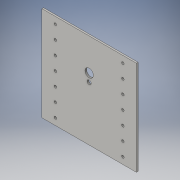
# Autodesk Inventor part: ClawPlate
Saved by Autodesk Inventor 2016 (Build 200138000, 138)
## iProperties
Created: 2016-01-25
Part Number: ClawPlate
Material: Generic
Document SubType Name: Modeling
Designer: Mentor1102
Density: 1 g/cm^3
Appearance: Default
Author: Mentor1102
Autodesk Inventor part; units mm, degrees
ref_plane "YZ Plane" through (0, 0, 0) normal (1, 0, 0) x (0, 1, 0)
ref_plane "XZ Plane" through (0, 0, 0) normal (0, 1, 0) x (-1, 0, 0)
ref_plane "XY Plane" through (0, 0, 0) normal (0, 0, 1) x (1, 0, 0)
sketch "Sketch1" plane through (0, 0, 0) normal (0, 0, 1) x (1, 0, 0)
  line L0 (0, 0) -> (177.8, 0)
  line L1 (177.8, 0) -> (177.8, 177.8)
  line L2 (177.8, 177.8) -> (0, 177.8)
  line L3 (0, 177.8) -> (0, 0)
  dimension "d0" = 177.8
  dimension "d1" = 177.8
  constraints: 8 end point, 2 parallel, 1 horizontal, 1 perpendicular
  measures "d0" distance of L2.end L1.end
  measures "d1" distance of L1.end L0.end
extrude "Extrusion1" add sketch "Sketch1" along normal blind 3.175
sketch "Sketch2" plane through (0, 0, 3.175) normal (0, 0, 1) x (1, 0, 0)
  line L0 (0, 0) -> (177.8, 0) projected
  line L1 (177.8, 0) -> (177.8, 177.8) projected
  line L2 (177.8, 177.8) -> (0, 177.8) construction
  line L3 (0, 177.8) -> (0, 0) projected
  line L4 (177.8, 177.8) -> (0, 177.8) construction
  line L5 (88.9, 177.8) -> (76.2, 177.8) construction
  line L6 (88.9, 177.8) -> (101.6, 177.8) construction
  line L7 (76.2, 177.8) -> (76.2, 127) construction
  line L8 (76.2, 127) -> (101.6, 127) construction
  line L9 (101.6, 177.8) -> (101.6, 127) construction
  line L10 (88.9, 127) -> (88.9, 107.95) construction
  circle A0 centre (88.9, 117.475) radius 9.525 construction
  circle A1 centre (88.9, 117.475) radius 7.874
  dimension "d4" = 12.7
  dimension "d5" = 12.7
  dimension "d6" = 50.8
  dimension "d7" = 19.05
  dimension "d8" = 15.748
  constraints: 12 end point, 3 midpoint, 3 vertical, 2 point on line, 1 centre point, 1 coincident, 1 perpendicular, 1 vertical alignment, 2 other
  measures "d4" distance of L5.start L5.end
  measures "d5" distance of L5.start L6.end
  measures "d6" distance of L5.end L7.end
  measures "d7" distance of L10.start L10.end
  measures "d8" diameter of A1
extrude "Extrusion2" cut sketch "Sketch2" against normal through all
sketch "Sketch3" plane through (0, 0, 3.175) normal (0, 0, 1) x (1, 0, 0)
  circle A0 centre (88.9, 117.475) radius 7.874 projected
  line L0 (0, 0) -> (177.8, 0) projected
  line L1 (177.8, 0) -> (177.8, 177.8) projected
  line L2 (177.8, 177.8) -> (0, 177.8) projected
  line L3 (0, 177.8) -> (0, 0) projected
  circle A1 centre (88.9, 117.475) radius 10.16 construction
  line L4 (88.9, 117.475) -> (88.9, 107.315) construction
  line L5 (88.9, 107.315) -> (88.9, 102.235) construction
  circle A2 centre (88.9, 102.235) radius 3.9116
  dimension "d11" = 20.32
  dimension "d12" = 5.08
  dimension "d13" = 7.8232
  constraints: 4 end point, 2 coincident, 2 vertical, 1 centre point, 1 vertical alignment, 2 other
  measures "d12" distance of L4.end L5.end
  measures "d13" diameter of A2
extrude "Extrusion3" cut sketch "Sketch3" against normal through all contours A2
sketch "Sketch4" plane through (0, 0, 3.175) normal (0, 0, 1) x (1, 0, 0)
  circle A0 centre (88.9, 102.235) radius 3.9116 projected
  circle A1 centre (88.9, 117.475) radius 7.874 projected
  line L0 (0, 0) -> (177.8, 0) projected
  line L1 (177.8, 0) -> (177.8, 177.8) projected
  line L2 (177.8, 177.8) -> (0, 177.8) construction
  line L3 (0, 177.8) -> (0, 0) projected
  line L4 (0, 177.8) -> (25.4, 177.8) construction
  line L5 (177.8, 177.8) -> (0, 177.8) construction
  line L6 (177.8, 177.8) -> (152.4, 177.8) construction
  line L7 (25.4, 177.8) -> (25.4, 152.4) construction
  line L8 (152.4, 177.8) -> (152.4, 152.4) construction
  circle A2 centre (25.4, 152.4) radius 2.3812
  circle A3 centre (152.4, 152.4) radius 2.3813
  line L9 (0, 165.1) -> (25.4, 165.1) construction
  line L10 (177.8, 165.1) -> (152.4, 165.1) construction
  line L11 (25.4, 165.1) -> (25.4, 139.7) construction
  line L12 (152.4, 165.1) -> (152.4, 139.7) construction
  circle A4 centre (25.4, 139.7) radius 2.3812
  line L13 (0, 152.4) -> (25.4, 152.4) construction
  line L14 (177.8, 152.4) -> (152.4, 152.4) construction
  line L15 (25.4, 152.4) -> (25.4, 127) construction
  line L16 (152.4, 152.4) -> (152.4, 127) construction
  circle A5 centre (25.4, 127) radius 2.3812
  line L17 (0, 139.7) -> (25.4, 139.7) construction
  line L18 (177.8, 139.7) -> (152.4, 139.7) construction
  line L19 (25.4, 139.7) -> (25.4, 114.3) construction
  line L20 (152.4, 139.7) -> (152.4, 114.3) construction
  circle A6 centre (25.4, 114.3) radius 2.3812
  line L21 (0, 127) -> (25.4, 127) construction
  line L22 (177.8, 127) -> (152.4, 127) construction
  line L23 (25.4, 127) -> (25.4, 101.6) construction
  line L24 (152.4, 127) -> (152.4, 101.6) construction
  circle A7 centre (25.4, 101.6) radius 2.3812
  line L25 (0, 114.3) -> (25.4, 114.3) construction
  line L26 (177.8, 114.3) -> (152.4, 114.3) construction
  line L27 (25.4, 114.3) -> (25.4, 88.9) construction
  line L28 (152.4, 114.3) -> (152.4, 88.9) construction
  circle A8 centre (25.4, 88.9) radius 2.3812
  line L29 (0, 101.6) -> (25.4, 101.6) construction
  line L30 (177.8, 101.6) -> (152.4, 101.6) construction
  line L31 (25.4, 101.6) -> (25.4, 76.2) construction
  line L32 (152.4, 101.6) -> (152.4, 76.2) construction
  circle A9 centre (25.4, 76.2) radius 2.3812
  line L33 (0, 88.9) -> (25.4, 88.9) construction
  line L34 (177.8, 88.9) -> (152.4, 88.9) construction
  line L35 (25.4, 88.9) -> (25.4, 63.5) construction
  line L36 (152.4, 88.9) -> (152.4, 63.5) construction
  circle A10 centre (25.4, 63.5) radius 2.3812
  line L37 (0, 76.2) -> (25.4, 76.2) construction
  line L38 (177.8, 76.2) -> (152.4, 76.2) construction
  line L39 (25.4, 76.2) -> (25.4, 50.8) construction
  line L40 (152.4, 76.2) -> (152.4, 50.8) construction
  circle A11 centre (25.4, 50.8) radius 2.3812
  line L41 (0, 63.5) -> (25.4, 63.5) construction
  line L42 (177.8, 63.5) -> (152.4, 63.5) construction
  line L43 (25.4, 63.5) -> (25.4, 38.1) construction
  line L44 (152.4, 63.5) -> (152.4, 38.1) construction
  circle A12 centre (25.4, 38.1) radius 2.3812
  line L45 (0, 50.8) -> (25.4, 50.8) construction
  line L46 (177.8, 50.8) -> (152.4, 50.8) construction
  line L47 (25.4, 50.8) -> (25.4, 25.4) construction
  line L48 (152.4, 50.8) -> (152.4, 25.4) construction
  circle A13 centre (25.4, 25.4) radius 2.3812
  line L49 (0, 38.1) -> (25.4, 38.1) construction
  line L50 (177.8, 38.1) -> (152.4, 38.1) construction
  line L51 (25.4, 38.1) -> (25.4, 12.7) construction
  line L52 (152.4, 38.1) -> (152.4, 12.7) construction
  circle A14 centre (25.4, 12.7) radius 2.3812
  circle A15 centre (152.4, 139.7) radius 2.3813
  circle A16 centre (152.4, 127) radius 2.3813
  circle A17 centre (152.4, 114.3) radius 2.3813
  circle A18 centre (152.4, 101.6) radius 2.3813
  circle A19 centre (152.4, 88.9) radius 2.3813
  circle A20 centre (152.4, 76.2) radius 2.3813
  circle A21 centre (152.4, 63.5) radius 2.3813
  circle A22 centre (152.4, 50.8) radius 2.3813
  circle A23 centre (152.4, 38.1) radius 2.3813
  circle A24 centre (152.4, 25.4) radius 2.3813
  circle A25 centre (152.4, 12.7) radius 2.3813
  circle A26 centre (25.4, 165.1) radius 2.3813
  circle A27 centre (152.4, 165.1) radius 2.3812
  dimension "d16" = 25.4
  dimension "d17" = 25.4
  dimension "d18" = 25.4
  dimension "d19" = 25.4
  dimension "d20" = 4.7625
  dimension "d21" = 4.7625
  dimension "d24" = 12.7
  dimension "d31" = 12.7
  dimension "d47" = 4.7625
  dimension "d48" = 4.7625
  constraints: 96 end point, 26 centre point, 17 coincident, 4 vertical, 2 point on line, 154 other
  measures "d16" distance of L2.end L4.end
  measures "d17" distance of L1.end L6.end
  measures "d18" distance of L4.end L7.end
  measures "d19" distance of L6.end L8.end
  measures "d20" diameter of A2
  measures "d21" diameter of A3
  measures "d24" distance of L4.end L9.end
  measures "d31" distance of A3.centre A15.centre
  measures "d47" diameter of A26
  measures "d48" diameter of A27
sketch "Sketch5" plane through (0, 0, 3.175) normal (0, 0, 1) x (1, 0, 0)
  circle A0 centre (88.9, 102.235) radius 3.9116 construction
  circle A1 centre (88.9, 117.475) radius 7.874 construction
  line L0 (0, 0) -> (177.8, 0) construction
  line L1 (177.8, 0) -> (177.8, 177.8) construction
  line L2 (177.8, 177.8) -> (0, 177.8) construction
  line L3 (0, 177.8) -> (0, 0) construction
  line L4 (177.8, 177.8) -> (0, 177.8) construction
  line L5 (88.9, 177.8) -> (76.2, 177.8) construction
  line L6 (88.9, 177.8) -> (101.6, 177.8) construction
  line L7 (76.2, 177.8) -> (25.4, 177.8)
  line L8 (101.6, 177.8) -> (152.4, 177.8)
  dimension "d43" = 12.7
  dimension "d44" = 12.7
  dimension "d45" = 50.8
  dimension "d46" = 50.8
  constraints: 8 end point, 4 point on line, 1 midpoint
  measures "d43" distance of L5.start L5.end
  measures "d44" distance of L5.start L6.end
  measures "d45" distance of L5.end L7.end
  measures "d46" distance of L6.end L8.end
hole "Hole2" at (25.4, 165.1, 3.175) at (152.4, 165.1, 3.175) at (25.4, 139.7, 3.175) at (25.4, 114.3, 3.175) at (25.4, 88.9, 3.175) at (25.4, 63.5, 3.175) at (25.4, 38.1, 3.175) at (25.4, 12.7, 3.175) at (152.4, 139.7, 3.175) at (152.4, 114.3, 3.175) at (152.4, 88.9, 3.175) at (152.4, 63.5, 3.175) at (152.4, 38.1, 3.175) at (152.4, 12.7, 3.175) direction (0, 0, -1) diameter 4.7625 end through all
body "Solid1"
